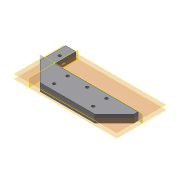
# Autodesk Inventor part: Cycl_soportePCB_A
Saved by Autodesk Inventor 2015 SP2 (Build 190223200, 223)
## iProperties
Created: 2015-04-21
Material: Genérico
Document SubType Name: Modeling
Designer: E.Beroiz
Density: 1 g/cm^3
Appearance: Valor por defecto
Description: Cycl_soportePCB_A
Author: E.Beroiz
Autodesk Inventor part; units mm, degrees
sketch "Boceto1" plane through (0, 0, 0) normal (0, 0, 1) x (1, 0, 0)
  line L0 (0, 0) -> (107, 0)
  line L1 (107, 0) -> (107, -5.5)
  line L2 (107, -5.5) -> (82, -30.4995)
  line L3 (82, -30.4995) -> (12, -30.4995)
  line L4 (12, -30.4995) -> (-13, -5.5)
  line L5 (-13, -5.5) -> (-13, 27)
  line L6 (-13, 27) -> (0, 27)
  line L7 (0, 27) -> (0, 0)
  dimension "d0" = 107
  dimension "d1" = 5.5
  dimension "d2" = 35.355
  dimension "d3" = 70
  dimension "d4" = 35.355
  dimension "d5" = 32.5
  dimension "d6" = 13
  dimension "d7" = 27
  constraints: 16 end point, 2 parallel, 2 perpendicular, 1 horizontal, 1 vertical, 1 vertical alignment
  measures "d0" distance of L0.start L0.end
  measures "d1" distance of L0.end L1.end
  measures "d2" distance of L1.end L2.end
  measures "d3" distance of L2.end L3.end
  measures "d4" distance of L3.end L4.end
  measures "d5" distance of L4.end L5.end
  measures "d6" distance of L5.end L6.end
  measures "d7" distance of L6.end L0.start
extrude "Extrusión1" add sketch "Boceto1" along normal blind 10
sketch "Boceto2" plane through (0, 0, 10) normal (0, 0, 1) x (1, 0, 0)
  circle A0 centre (22, -5.4995) radius 1.89
  circle A1 centre (47, -5.4995) radius 1.89
  circle A2 centre (72, -5.4995) radius 1.89
  circle A3 centre (-5.5, 12) radius 1.89
  circle A4 centre (22, -22.7495) radius 1.89
  circle A5 centre (72, -22.7495) radius 1.89
  line L0 (12, -30.4995) -> (82, -30.4995) projected
  line L1 (-13, 27) -> (-13, -5.5) projected
  line L2 (0, 27) -> (-13, 27) projected
  line L3 (0, 27) -> (0, 0) projected
  dimension "d10" = 3.78
  dimension "d11" = 3.78
  dimension "d12" = 3.78
  dimension "d13" = 3.78
  dimension "d14" = 3.78
  dimension "d15" = 3.78
  dimension "d16" = 25
  dimension "d17" = 25
  dimension "d18" = 17.25
  dimension "d19" = 7.75
  dimension "d20" = 35
  dimension "d21" = 15
  dimension "d22" = 5.5
  constraints: 6 centre point, 3 horizontal alignment, 2 vertical alignment
  measures "d10" diameter of A0
  measures "d11" diameter of A1
  measures "d12" diameter of A2
  measures "d13" diameter of A3
  measures "d14" diameter of A4
  measures "d15" diameter of A5
  measures "d16" distance of A0.centre A1.centre
  measures "d17" distance of A2.centre A1.centre
  measures "d18" distance of A5.centre A2.centre
  measures "d19" distance from line of L0 A5.centre
  measures "d20" distance from line of L1 A4.centre
  measures "d21" distance from line of L2 A3.centre
  measures "d22" distance from line of L3 A3.centre
extrude "Extrusión2" cut sketch "Boceto2" against normal through all
sketch "Boceto3" plane through (0, 0, 0) normal (0, 0, -1) x (-1, 0, 0)
  circle A0 centre (-72, -22.7495) radius 1.89 projected
  circle A1 centre (-22, -22.7495) radius 1.89 projected
  circle A2 centre (-72, -22.7495) radius 3.6
  circle A3 centre (-22, -22.7495) radius 3.6
  point P0 (0, 0)
  dimension "d25" = 7.2
  dimension "d26" = 7.2
  constraints: 2 centre point, 2 coincident
  measures "d25" diameter of A2
  measures "d26" diameter of A3
extrude "Extrusión3" cut sketch "Boceto3" against normal blind 2.79
ref_plane "Plano de trabajo1" through (0, 0, 5.61) normal (0, 0, 1) x (1, 0, 0)
sketch "Boceto4" plane through (0, 0, 5.61) normal (0, 0, 1) x (1, 0, 0)
  circle A0 centre (-5.5, 12) radius 1.89 projected
  circle A1 centre (22, -5.4995) radius 1.89 projected
  circle A2 centre (47, -5.4995) radius 1.89 projected
  circle A3 centre (72, -5.4995) radius 1.89 projected
  line L0 (0, 27) -> (0, 0) projected
  line L1 (0, 15.1175) -> (-7.3, 15.1175)
  line L2 (-7.3, 15.1175) -> (-9.1003, 12)
  line L3 (-9.1003, 12) -> (-7.3, 8.8825)
  line L4 (-7.3, 8.8825) -> (0, 8.8825)
  line L5 (0, 15.1175) -> (0, 8.8825)
  line L6 (22, -9.1003) -> (18.8825, -7.3)
  line L7 (18.8825, -7.3) -> (18.8825, 0)
  line L8 (0, 0) -> (107, 0) projected
  line L9 (22, -9.1003) -> (25.1175, -7.3)
  line L10 (25.1175, -7.3) -> (25.1175, 0)
  line L11 (25.1175, 0) -> (18.8825, 0)
  point P0 (0, 12)
  point P1 (22, 0)
  dimension "d30" = 7.3
  dimension "d31" = 6.235
  dimension "d32" = 3.6
  dimension "d33" = 6.235
  dimension "d34" = 3.6
  dimension "d35" = 7.3
  constraints: 20 end point, 4 point on line, 3 equal length, 2 horizontal alignment, 2 midpoint, 2 parallel, 2 perpendicular, 2 vertical alignment, 1 collinear, 1 vertical
  measures "d30" distance of L1.start L1.end
  measures "d31" distance between parallel lines of L4 L1
  measures "d32" distance of L1.end L2.end
  measures "d33" distance between parallel lines of L7 L10
  measures "d34" distance of L6.start L9.end
  measures "d35" distance of L9.end L10.end
extrude "Extrusión4" cut sketch "Boceto4" against normal blind 3 contours L8 L10 L9 L6 L7 | L0 L4 L3 L2 L1
pattern_linear "Patrón rectangular1" count 3 spacing -25 along (-1, 0, 0) of "Extrusión4"
sketch "Boceto5" plane through (0, 0, 0) normal (0, 0, -1) x (-1, 0, 0)
  line L0 (-98, 0) -> (-98, -4)
  line L1 (-98, -4) -> (4, -4)
  line L2 (4, -4) -> (4, 27)
  line L3 (13, 27) -> (0, 27) projected
  line L4 (0, 27) -> (4, 27)
  line L5 (0, 27) -> (0, 0)
  line L6 (0, 0) -> (0, 27) projected
  line L7 (0, 0) -> (-98, 0)
  line L8 (-107, 0) -> (-107, -5.5) projected
  line L9 (13, -5.5) -> (13, 27) projected
  dimension "d41" = 4
  dimension "d42" = 9
  dimension "d43" = 9
  constraints: 12 end point, 3 perpendicular, 2 collinear, 1 point on line, 1 vertical
  measures "d41" distance of L0.start L0.end
  measures "d42" distance between parallel lines of L8 L0
  measures "d43" distance between parallel lines of L9 L2
extrude "Extrusión5" cut sketch "Boceto5" against normal blind 0.8
